PLATE_HV_BACK (Autodesk Fusion 360 design; units mm, degrees)
Autodesk Fusion 360 part; units mm, degrees
sketch "Esquisse1" plane through (0, 0, 0) normal (0, 0, 1) x (1, 0, 0)
  line L0 (75, 23) -> (-75, 23)
  line L1 (-75, 23) -> (-75, -23)
  line L2 (-75, -23) -> (75, -23)
  line L3 (75, -23) -> (75, 23)
  line L4 (75, 23) -> (-75, -23) construction
  line L5 (-75, 23) -> (75, -23) construction
  line L6 (78, -20) -> (-78, -20)
  line L7 (-78, -20) -> (-78, 20)
  line L8 (-78, 20) -> (78, 20)
  line L9 (78, 20) -> (78, -20)
  line L10 (78, -20) -> (-78, 20) construction
  line L11 (-78, -20) -> (78, 20) construction
  dimension "d1" = 150
  dimension "d2" = 156
  dimension "d3" = 40
  dimension "d4" = 46
  constraint horizontal L0
  constraint perpendicular L0 L1
  constraint parallel L0 L2
  constraint parallel L1 L3
  constraint coincident L4 origin
  constraint coincident L5 origin
  constraint horizontal L6
  constraint perpendicular L6 L7
  constraint parallel L6 L8
  constraint parallel L7 L9
  constraint coincident L10 origin
  constraint coincident L11 origin
  measures "d1" distance of L0.start L0.end
  measures "d2" distance of L7.end L8.end
  measures "d3" distance of L6.end L7.end
  measures "d4" distance of L0.end L1.end
extrude "Extrusion1" add sketch "Esquisse1" along normal blind 3
equation "d2 = d1 + ( 2 * 3 ) * 1 mm"
equation "d4 = d3 + ( 2 * 3 ) * 1 mm"
equation "Transfo_notch_larg_Ref = 1.6 mm" comment "epaisseur des encoches du transfo"
equation "Trasnfo_notch_long_Ref = 4 mm" comment "Longueurs des encoches du transfo"
equation "Transfo_Dist_Larg_2_notchs_Ref = 11.9 mm" comment "Distance entre deux encoches (largeur)"
equation "Transfo_Dist_Long_2_nothcs_Ref = 39 mm - ( 2 * 1.6 ) * 1 mm" comment "Distance (longueur) entre deux encoches"
equation "Transfo_Hole_Diam_Ref = 3.7 mm" comment "Diamètre des trous du transfo"
equation "Transfo_Dist_2_Hole_Ref = 16.7 mm" comment "Distance entre les centres des trous du transfo"
equation "Transfo_Dist_Notch_Hole_Ref = 69.2 mm" comment "Distance (minimal) entre les encoches et les trous"
